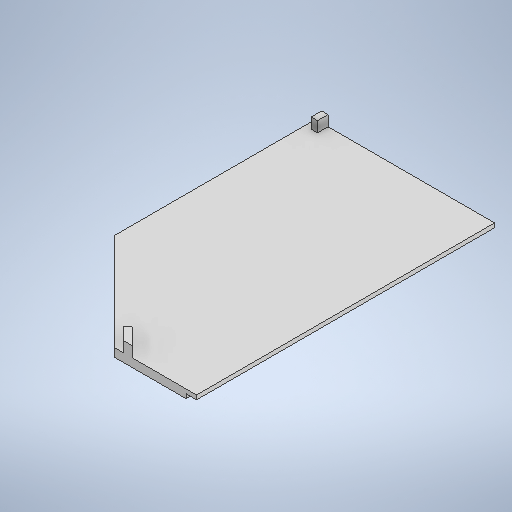
# Autodesk Inventor part: side_wall
Saved by Autodesk Inventor 2026.1 (Build 301233000, 233)
## iProperties
Created: 2026-08-11
Part Number: side_wall
Material: Generic
Document SubType Name: Modeling
Designer: rowan
Density: 1 g/cm^3
Appearance: Default
Author: rowan
Autodesk Inventor part; units mm, degrees
ref_plane "YZ Plane" through (0, 0, 0) normal (1, 0, 0) x (0, 1, 0)
ref_plane "XZ Plane" through (0, 0, 0) normal (0, 1, 0) x (-1, 0, 0)
ref_plane "XY Plane" through (0, 0, 0) normal (0, 0, 1) x (1, 0, 0)
sketch "Sketch1" plane through (0, 0, 0) normal (0, 1, 0) x (-1, 0, 0)
  line L0 (80, -141.4) -> (0, -141.4)
  line L1 (0, -141.4) -> (0, 0)
  line L2 (0, 0) -> (34.0381, 0)
  line L3 (34.0381, 0) -> (80, -45.9619)
  line L4 (80, -45.9619) -> (80, -141.4)
  dimension "d0" = 80
  dimension "d1" = 141.4
  dimension "d7" = 135
  dimension "d8" = 65
  constraints: 10 end point, 2 perpendicular, 1 horizontal, 1 parallel
  measures "d0" distance of L0.start L0.end
  measures "d1" distance of L0.end L1.end
  measures "d7" angle of L3 L2
  measures "d8" distance of L2.end L3.end
extrude "Extrusion1" add sketch "Sketch1" along normal blind 4
sketch "Sketch2" plane through (0, 4, 0) normal (0, 1, 0) x (1, 0, 0)
  line L0 (0, 0) -> (0, 141.4) projected
  line L1 (0, 0) -> (5, 0)
  line L2 (5, 0) -> (5, 141.4)
  line L3 (5, 141.4) -> (0, 141.4)
  line L4 (0, 141.4) -> (0, 0)
  point P0 (0, 141.4)
  dimension "d4" = 5
  constraints: 8 end point, 2 parallel, 1 horizontal, 1 perpendicular
  measures "d4" distance of L0.start L1.end
extrude "Extrusion2" add sketch "Sketch2" against normal blind 2
sketch "Sketch3" plane through (0, 4, 0) normal (0, 1, 0) x (1, 0, 0)
  line L0 (-34.0381, 0) -> (5, 0) projected
  line L1 (-29.7954, 0) -> (-35.4523, 5.6569)
  line L2 (-80, 45.9619) -> (-34.0381, 0) projected
  line L3 (-29.7954, 0) -> (-25.5528, 0)
  line L4 (-25.5528, 0) -> (-33.331, 7.7782)
  line L5 (-33.331, 7.7782) -> (-35.4523, 5.6569)
  line L6 (-77, 136.4) -> (-74, 136.4)
  line L7 (-74, 136.4) -> (-74, 141.4)
  line L8 (-74, 141.4) -> (-77, 141.4)
  line L9 (-77, 141.4) -> (-77, 136.4)
  line L10 (-80, 141.4) -> (-80, 45.9619) projected
  line L11 (5, 141.4) -> (-80, 141.4) projected
  point P0 (0, 0)
  dimension "d9" = 8
  dimension "d10" = 3
  dimension "d15" = 3
  dimension "d16" = 5
  dimension "d17" = 3
  constraints: 16 end point, 3 parallel, 3 perpendicular, 2 point on line, 1 collinear, 1 equal length, 1 horizontal
  measures "d9" distance of L1.start L1.end
  measures "d10" distance between parallel lines of L1 L2
  measures "d15" distance of L4.end L1.end
  measures "d16" distance of L8.end L6.start
  measures "d17" distance between parallel lines of L10 L9
extrude "Extrusion3" add sketch "Sketch3" along normal blind 5
body "Solid1"
